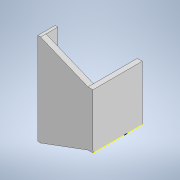
# Autodesk Inventor part: gira
Saved by Autodesk Inventor 2020 (Build 240168000, 168)
## iProperties
Created: 2022-10-31
Part Number: gira
Material: Generic
Document SubType Name: Modeling
Designer: super
Density: 1 g/cm^3
Appearance: Default
Author: super
Autodesk Inventor part; units mm, degrees
ref_plane "YZ Plane" through (0, 0, 0) normal (1, 0, 0) x (0, 1, 0)
ref_plane "XZ Plane" through (0, 0, 0) normal (0, 1, 0) x (-1, 0, 0)
ref_plane "XY Plane" through (0, 0, 0) normal (0, 0, 1) x (1, 0, 0)
ref_plane "Work Plane1" through (-84.5679, -177.7614, 10.4079) normal (0.999999, 0.0014131, 0) x (0.0014131, -0.999999, 0)
sketch "Sketch1" plane through (-84.5679, -177.7614, 10.4079) normal (0.999999, 0.0014131, 0) x (0.0014131, -0.999999, 0)
  line L0 (9.6295, -13.989) -> (-157.4911, -13.989)
  line L1 (-157.4911, -13.989) -> (-157.4911, 7.4134)
  line L2 (-157.4911, 7.4134) -> (9.6295, 7.4134)
  line L3 (9.6295, 7.4134) -> (9.6295, -13.989)
  point P0 (-177.6417, 10.4079)
  constraints: 8 end point, 2 parallel, 1 horizontal, 1 perpendicular
extrude "Extrusion1" add sketch "Sketch1" along normal blind 5
ref_plane "Work Plane2" through (-84.6723, -103.8307, 24.3968) normal (-0.0014131, 0.999999, 0) x (0.999999, 0.0014131, 0)
sketch "Sketch3" plane through (-84.5543, -187.3909, 24.3968) normal (0, 0, 1) x (0.999999, 0.0014131, 0)
  line L0 (0, 0) -> (5, 0)
  line L1 (5, 0) -> (91.2544, 31.8306)
  line L2 (91.2544, 31.8306) -> (100.3623, 31.8306)
  line L3 (100.3623, 31.8306) -> (100.3623, 131.4706)
  line L4 (100.3623, 131.4706) -> (91.2544, 131.4706)
  line L5 (5, 0) -> (5, 167.1206) projected
  line L6 (91.2544, 131.4706) -> (5, 167.1206)
  line L7 (0, 0) -> (0, 167.1206) projected
  line L8 (5, 167.1206) -> (0, 167.1206)
  line L9 (0, 167.1206) -> (0, 0)
  point P0 (84.819, 187.2712)
  constraints: 16 end point, 3 perpendicular, 2 parallel, 1 horizontal
extrude "Extrusion2" add sketch "Sketch3" along normal blind 10
sketch "Sketch4" plane through (-84.5543, -187.3909, 24.3968) normal (0, 0, -1) x (-0.999999, -0.0014131, 0)
  line L0 (-100.3623, 131.4706) -> (-91.2544, 131.4706) projected
  line L1 (-91.2544, 31.8306) -> (-100.3623, 31.8306) projected
  line L2 (-100.3623, 131.4706) -> (-91.2544, 131.4706)
  line L3 (-91.2544, 131.4706) -> (-91.2544, 31.8306)
  line L4 (-91.2544, 31.8306) -> (-100.3623, 31.8306)
  line L5 (-100.3623, 31.8306) -> (-100.3623, 131.4706)
  point P0 (-84.819, 187.2712)
  point P1 (-100.3623, 31.8306)
  point P2 (-91.2544, 131.4706)
  constraints: 8 end point, 2 parallel, 1 horizontal, 1 perpendicular
extrude "Extrusion3" add sketch "Sketch4" along normal blind 80
sketch "Sketch6" plane through (15.7629, -155.4186, -55.6032) normal (0.0014131, -0.999999, 0) x (0.999999, 0.0014131, 0)
  line L0 (0, 0) -> (0, 90) projected
  line L1 (0, 28.5548) -> (0, 34.1867)
  line L2 (0, 34.1867) -> (-17.3106, 34.1867)
  line L3 (-17.3106, 34.1867) -> (-17.3106, 28.5548)
  line L4 (-17.3106, 28.5548) -> (0, 28.5548)
  point P0 (-15.5433, 55.6032)
  constraints: 8 end point, 2 parallel, 2 point on line, 1 perpendicular
extrude "Extrusion5" add sketch "Sketch6" along normal blind 100
sketch "Sketch7" plane through (6.6551, -155.4314, -27.0484) normal (0, 0, -1) x (-0.999999, -0.0014131, 0)
  line L0 (8.2028, 0) -> (0, 14.7244)
  line L1 (0, 99.6401) -> (0, 0) projected
  line L2 (8.2028, 0) -> (0, 0) projected
  line L3 (0, 0) -> (8.2028, 0)
  constraints: 4 end point, 1 collinear, 1 point on line
extrude "Extrusion6" add sketch "Sketch7" against normal blind 10
ref_plane "Work Plane3" through (15.6925, -105.5986, 34.3968) normal (-0.0014131, 0.999999, 0) x (0.999999, 0.0014131, 0)
mirror "Mirror1" about plane through (15.6925, -105.5986, 34.3968) normal (-0.0014131, 0.999999, 0) of "Extrusion5", "Extrusion6"
body "Solid1"
